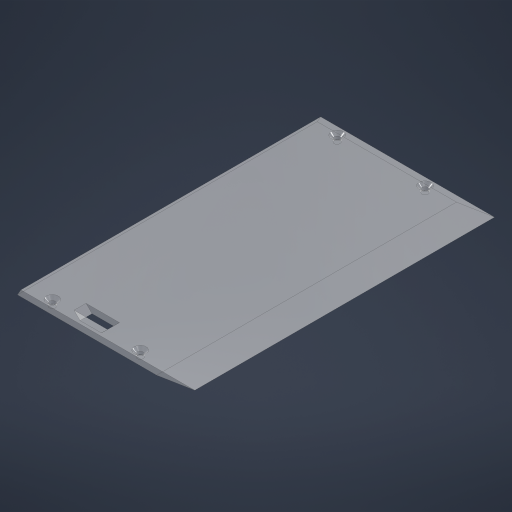
# Autodesk Inventor part: porywa
Saved by Autodesk Inventor 2024 (Build 280153000, 153)
## iProperties
Created: 2024-05-25
Part Number: porywa
Material: Polycarbonate, Clear
Document SubType Name: Modeling
Designer: Adam
Density: 1.2 g/cm^3
Appearance: Polycarbonate - Clear
Author: Adam
Autodesk Inventor part; units mm, degrees
ref_plane "YZ Plane" through (0, 0, 0) normal (1, 0, 0) x (0, 1, 0)
ref_plane "XZ Plane" through (0, 0, 0) normal (0, 1, 0) x (-1, 0, 0)
ref_plane "XY Plane" through (0, 0, 0) normal (0, 0, 1) x (1, 0, 0)
sketch "Sketch1" plane through (0, 0, 0) normal (0, 0, 1) x (1, 0, 0)
  line L0 (-24.865, 1.7403) -> (-26.0197, -0.2597)
  line L1 (-26.0197, -0.2597) -> (20.4267, -0.2597)
  line L2 (-24.865, 1.7403) -> (33.135, 1.7403)
  line L3 (33.135, 1.7403) -> (20.4267, -0.2597)
  point P0 (0, 0)
  dimension "d0" = 58
  constraints: 8 end point, 1 point on line
  measures "d0" distance of L0.start L2.end
extrude "Extrusion1" add sketch "Sketch1" along normal blind 100
sketch "Sketch2" plane through (-24.865, 1.7403, 0) normal (0, 1, 0) x (1, 0, 0)
  line L0 (-1.1547, 0) -> (45.2917, 0) projected
  line L1 (58, -100) -> (0, -100) projected
  line L2 (0, 0) -> (0, -100) projected
  line L3 (45.2917, 0) -> (45.2917, -100) projected
  point P0 (24.865, 0)
  point P1 (8, -2.5)
  point P2 (37.2917, -2.5)
  point P3 (8, -97.5)
  point P4 (37.2917, -97.5)
  dimension "d3" = 2.5
  dimension "d4" = 2.5
  dimension "d5" = 2.5
  dimension "d6" = 2.5
  dimension "d7" = 8
  dimension "d8" = 8
  dimension "d9" = 8
  dimension "d10" = 8
  measures "d3" distance from line of L0 point (8, -2.5)
  measures "d4" distance from line of L0 point (37.292, -2.5)
  measures "d5" distance from line of L1 point (8, -97.5)
  measures "d6" distance from line of L1 point (37.292, -97.5)
  measures "d7" distance from line of point (8, -2.5) L2
  measures "d8" distance from line of L3 point (37.292, -2.5)
  measures "d9" distance from line of L3 point (37.292, -97.5)
  measures "d10" distance from line of L2 point (8, -97.5)
hole "Hole1" at (-16.865, 1.7403, 2.5) at (12.4267, 1.7403, 2.5) at (-16.865, 1.7403, 97.5) at (12.4267, 1.7403, 97.5) direction (0, -1, 0) diameter 2 end through all
chamfer "Chamfer1" distance 1 angle 45 4 edges at (-16.865, 1.7403, 1.5) (12.4267, 1.7403, 1.5) (-16.865, 1.7403, 96.5) (12.4267, 1.7403, 96.5) measured on face at (12.4267, 1.7403, 1) measured on face at (12.4267, 1.7403, 96) measured on face at (-16.865, 1.7403, 96) measured on face at (-16.865, 1.7403, 1)
sketch "Sketch3" plane through (-24.865, 1.7403, 0) normal (0, 1, 0) x (1, 0, 0)
  line L0 (16.7348, -93) -> (23.8856, -93)
  line L1 (23.8856, -93) -> (23.8856, -97)
  line L2 (23.8856, -97) -> (16.7348, -97)
  line L3 (16.7348, -97) -> (16.7348, -93)
  point P0 (24.865, 0)
  point P1 (16.7856, -97)
  point P2 (23.8348, -93)
  constraints: 8 end point, 2 parallel, 1 horizontal, 1 perpendicular
extrude "Extrusion2" cut sketch "Sketch3" against normal through all
chamfer "Chamfer2" distance 2 angle 45 2 edges at (-8.1302, 1.7403, 95) (-0.9794, 1.7403, 95) measured on face at (-8.6302, 1.7403, 95) measured on face at (-0.4794, 1.7403, 95)
body "Solid1"
